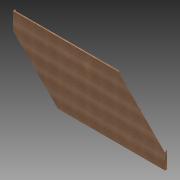
# Autodesk Inventor part: Base
Saved by Autodesk Inventor 2014 SP1 (Build 180222100, 222)
## iProperties
Created: 2015-03-28
Part Number: Base
Material: Wood (Birch)
Document SubType Name: Modeling
Designer: tuleu
Density: 0.55 g/cm^3
Appearance: Birch - Natural Polished
Author: tuleu
Autodesk Inventor part; units mm, degrees
ref_plane "YZ Plane" through (0, 0, 0) normal (1, 0, 0) x (0, 1, 0)
ref_plane "XZ Plane" through (0, 0, 0) normal (0, 1, 0) x (-1, 0, 0)
ref_plane "XY Plane" through (0, 0, 0) normal (0, 0, 1) x (1, 0, 0)
sketch "Sketch1" plane through (0, 0, 0) normal (0, 1, 0) x (-1, 0, 0)
  line L0 (1400, 575) -> (-1400, 575)
  line L1 (-1400, 575) -> (-1400, -575)
  line L2 (-1400, -575) -> (1400, -575)
  line L3 (1400, -575) -> (1400, 575)
  line L4 (0, -575) -> (0, 575)
  line L5 (-1400, 0) -> (1400, 0)
  point P0 (0, 0)
  dimension "d0" = 2800
  dimension "d1" = 1150
  constraints: 12 end point, 6 midpoint, 2 parallel, 1 horizontal, 1 perpendicular
  measures "d0" distance of L1.end L2.end
  measures "d1" distance of L2.end L0.start
extrude "Extrusion1" add sketch "Sketch1" along normal blind 19
sketch "Sketch2" plane through (0, 19, 0) normal (0, 1, 0) x (1, 0, 0)
  line L0 (1400, 575) -> (-1400, 575) projected
  line L1 (-1400, 575) -> (-1400, -575) projected
  line L2 (-1400, -575) -> (1400, -575) projected
  line L3 (1400, -575) -> (1400, 575) projected
  line L4 (-1385, -575) -> (-1385, 575)
  line L5 (1385, 575) -> (1385, -575)
  line L6 (-1385, -575) -> (-1400, -575)
  line L7 (-1400, 575) -> (-1400, -575)
  line L8 (1400, 575) -> (1400, -575)
  line L9 (1400, -575) -> (1385, -575)
  line L10 (-1400, 575) -> (-1385, 575)
  line L11 (1385, 575) -> (1400, 575)
  point P0 (0, 0)
  dimension "d4" = 15
  dimension "d5" = 15
  constraints: 16 end point, 4 perpendicular, 3 collinear, 2 point on line, 1 parallel
  measures "d4" distance between parallel lines of L1 L4
  measures "d5" distance between parallel lines of L3 L5
extrude "Extrusion2" add sketch "Sketch2" along normal blind 19 contours L3 L2 L5 L0 | L4 L2 L1 L0
sketch "Sketch4" plane through (0, 19, 0) normal (0, 1, 0) x (1, 0, 0)
  line L0 (-1385, 575) -> (-1385, -575) projected
  line L1 (-1385, -575) -> (1385, -575) projected
  line L2 (1385, -575) -> (1385, 575) projected
  line L3 (1385, 575) -> (-1385, 575) projected
  line L4 (-1255, -225) -> (-1309.8, -225) projected
  line L5 (-1177.5, 175) -> (-1232.3, 175) projected
  line L6 (-1275, 475) -> (-1385, 475) projected
  line L7 (-1165, 475) -> (-1270, 475) projected
  line L8 (-1060, 475) -> (-1160, 475) projected
  line L9 (-950, 475) -> (-1055, 475) projected
  line L10 (-835, 475) -> (-945, 475) projected
  line L11 (-735, 475) -> (-830, 475) projected
  line L12 (-625, 475) -> (-730, 475) projected
  line L13 (-520, 475) -> (-620, 475) projected
  line L14 (-410, 475) -> (-515, 475) projected
  line L15 (-305, 475) -> (-405, 475) projected
  line L16 (-195, 475) -> (-300, 475) projected
  line L17 (-95, 475) -> (-190, 475) projected
  line L18 (20, 475) -> (-90, 475) projected
  line L19 (130, 475) -> (25, 475) projected
  line L20 (235, 475) -> (135, 475) projected
  line L21 (345, 475) -> (240, 475) projected
  line L22 (460, 475) -> (350, 475) projected
  line L23 (560, 475) -> (465, 475) projected
  line L24 (670, 475) -> (565, 475) projected
  line L25 (775, 475) -> (675, 475) projected
  line L26 (885, 475) -> (780, 475) projected
  line L27 (990, 475) -> (890, 475) projected
  line L28 (1100, 475) -> (995, 475) projected
  line L29 (1200, 475) -> (1105, 475) projected
  line L30 (1385, 475) -> (1205, 475) projected
  line L31 (0, 575) -> (0, 475)
  line L32 (-1385, 525) -> (1385, 525)
  line L33 (-1332.5, 542.5) -> (1297.5, 542.5)
  line L34 (-1330, 475) -> (-1330, -575)
  line L35 (-1217.5, 475) -> (-1217.5, -575)
  line L36 (-1110, 475) -> (-1110, -575)
  line L37 (-1002.5, 475) -> (-1002.5, -575)
  line L38 (-890, 475) -> (-890, -575)
  line L39 (-782.5, 475) -> (-782.5, -575)
  line L40 (-677.5, 475) -> (-677.5, -575)
  line L41 (-570, 475) -> (-570, -575)
  line L42 (-462.5, 475) -> (-462.5, -575)
  line L43 (-355, 475) -> (-355, -575)
  line L44 (-247.5, 475) -> (-247.5, -575)
  line L45 (-142.5, 475) -> (-142.5, -575)
  line L46 (-35, 475) -> (-35, -575)
  line L47 (77.5, 475) -> (77.5, -575)
  line L48 (185, 475) -> (185, -575)
  line L49 (292.5, 475) -> (292.5, -575)
  line L50 (405, 475) -> (405, -575)
  line L51 (512.5, 475) -> (512.5, -575)
  line L52 (617.5, 475) -> (617.5, -575)
  line L53 (725, 475) -> (725, -575)
  line L54 (832.5, 475) -> (832.5, -575)
  line L55 (940, 475) -> (940, -575)
  line L56 (1047.5, 475) -> (1047.5, -575)
  line L57 (1152.5, 475) -> (1152.5, -575)
  line L58 (1295, 475) -> (1295, -575)
  line L59 (-780, 507.5) -> (-780, -195)
  line L60 (-780, -205) -> (-785, -205)
  line L61 (-785, -205) -> (-785, 507.5)
  line L62 (-675, 507.5) -> (-675, 205)
  line L63 (-675, 195) -> (-680, 195)
  line L64 (-680, 205) -> (-680, 507.5)
  line L65 (-567.5, 507.5) -> (-567.5, -195)
  line L66 (-567.5, -205) -> (-572.5, -205)
  line L67 (-572.5, -195) -> (-572.5, 507.5)
  line L68 (-460, 507.5) -> (-460, 205)
  line L69 (-460, 195) -> (-465, 195)
  line L70 (-465, 205) -> (-465, 507.5)
  line L71 (-352.5, 507.5) -> (-352.5, -195)
  line L72 (-352.5, -205) -> (-357.5, -205)
  line L73 (-357.5, -195) -> (-357.5, 507.5)
  line L74 (-245, 507.5) -> (-245, 205)
  line L75 (-245, 195) -> (-250, 195)
  line L76 (-250, 205) -> (-250, 507.5)
  line L77 (-140, 507.5) -> (-140, -205)
  line L78 (-140, -205) -> (-145, -205)
  line L79 (-145, -195) -> (-145, 507.5)
  line L80 (-1327.5, 507.5) -> (-1327.5, -195)
  line L81 (-1327.5, -205) -> (-1332.5, -205)
  line L82 (-1332.5, -205) -> (-1332.5, 542.5)
  line L83 (-1215, 507.5) -> (-1215, 205)
  line L84 (-1215, 195) -> (-1220, 195)
  line L85 (-1220, 205) -> (-1220, 507.5)
  line L86 (-1107.5, 507.5) -> (-1107.5, -195)
  line L87 (-1107.5, -205) -> (-1112.5, -205)
  line L88 (-1112.5, -195) -> (-1112.5, 507.5)
  line L89 (-1000, 507.5) -> (-1000, 205)
  line L90 (-1000, 195) -> (-1005, 195)
  line L91 (-1005, 205) -> (-1005, 507.5)
  line L92 (-887.5, 507.5) -> (-887.5, -205)
  line L93 (-887.5, -205) -> (-892.5, -205)
  line L94 (-892.5, -195) -> (-892.5, 507.5)
  line L95 (-32.5, 507.5) -> (-32.5, -195)
  line L96 (-32.5, -205) -> (-37.5, -205)
  line L97 (-37.5, -205) -> (-37.5, 507.5)
  line L98 (80, 507.5) -> (80, 205)
  line L99 (80, 195) -> (75, 195)
  line L100 (75, 205) -> (75, 507.5)
  line L101 (-1220, 507.5) -> (-1327.5, 507.5)
  line L102 (-1112.5, 507.5) -> (-1215, 507.5)
  line L103 (-1005, 507.5) -> (-1107.5, 507.5)
  line L104 (-892.5, 507.5) -> (-1000, 507.5)
  line L105 (-785, 507.5) -> (-887.5, 507.5)
  line L106 (-680, 507.5) -> (-780, 507.5)
  line L107 (-572.5, 507.5) -> (-675, 507.5)
  line L108 (-465, 507.5) -> (-567.5, 507.5)
  line L109 (-357.5, 507.5) -> (-460, 507.5)
  line L110 (-250, 507.5) -> (-352.5, 507.5)
  line L111 (-145, 507.5) -> (-245, 507.5)
  line L112 (-37.5, 507.5) -> (-140, 507.5)
  line L113 (75, 507.5) -> (-32.5, 507.5)
  line L114 (-1385, -205) -> (1385, -205)
  line L115 (187.5, 507.5) -> (187.5, -195)
  line L116 (187.5, -205) -> (182.5, -205)
  line L117 (182.5, -195) -> (182.5, 507.5)
  line L118 (295, 507.5) -> (295, 205)
  line L119 (295, 195) -> (290, 195)
  line L120 (290, 205) -> (290, 507.5)
  line L121 (407.5, 507.5) -> (407.5, -205)
  line L122 (407.5, -205) -> (402.5, -205)
  line L123 (402.5, -195) -> (402.5, 507.5)
  line L124 (515, 507.5) -> (515, -195)
  line L125 (515, -205) -> (510, -205)
  line L126 (510, -205) -> (510, 507.5)
  line L127 (620, 507.5) -> (620, 205)
  line L128 (620, 195) -> (615, 195)
  line L129 (615, 205) -> (615, 507.5)
  line L130 (727.5, 507.5) -> (727.5, -195)
  line L131 (727.5, -205) -> (722.5, -205)
  line L132 (722.5, -205) -> (722.5, 507.5)
  line L133 (835, 507.5) -> (835, 205)
  line L134 (835, 195) -> (830, 195)
  line L135 (830, 205) -> (830, 507.5)
  line L136 (942.5, 507.5) -> (942.5, -195)
  line L137 (942.5, -205) -> (937.5, -205)
  line L138 (937.5, -195) -> (937.5, 507.5)
  line L139 (1050, 507.5) -> (1050, 205)
  line L140 (1050, 195) -> (1045, 195)
  line L141 (1045, 205) -> (1045, 507.5)
  line L142 (1155, 507.5) -> (1155, -205)
  line L143 (1155, -205) -> (1150, -205)
  line L144 (1150, -195) -> (1150, 507.5)
  line L145 (182.5, 507.5) -> (80, 507.5)
  line L146 (290, 507.5) -> (187.5, 507.5)
  line L147 (402.5, 507.5) -> (295, 507.5)
  line L148 (510, 507.5) -> (407.5, 507.5)
  line L149 (615, 507.5) -> (515, 507.5)
  line L150 (722.5, 507.5) -> (620, 507.5)
  line L151 (830, 507.5) -> (727.5, 507.5)
  line L152 (937.5, 507.5) -> (835, 507.5)
  line L153 (1045, 507.5) -> (942.5, 507.5)
  line L154 (1150, 507.5) -> (1050, 507.5)
  line L155 (1292.5, 507.5) -> (1155, 507.5)
  line L156 (1297.5, 542.5) -> (1297.5, -195)
  line L157 (1297.5, -205) -> (1292.5, -205)
  line L158 (1292.5, -195) -> (1292.5, 507.5)
  line L159 (-1385, 195) -> (1385, 195)
  line L160 (-1327.5, -195) -> (-1262.5, -195)
  line L161 (-1262.5, -195) -> (-1262.5, -205)
  line L162 (-1262.5, -205) -> (-1327.5, -205)
  line L163 (-1280.2, -200) -> (-1280.2, -225) projected
  line L164 (-1309.8, -250) -> (-1309.8, -200) projected
  line L165 (-1309.8, -200) -> (-1280.2, -200)
  line L166 (-1295, -200) -> (-1295, -195)
  line L167 (-1220, 205) -> (-1245, 205)
  line L168 (-1245, 205) -> (-1245, 195)
  line L169 (-1245, 195) -> (-1220, 195)
  line L170 (-1215, 205) -> (-1190, 205)
  line L171 (-1190, 205) -> (-1190, 195)
  line L172 (-1190, 195) -> (-1215, 195)
  line L173 (-1112.5, -195) -> (-1137.5, -195)
  line L174 (-1137.5, -195) -> (-1137.5, -205)
  line L175 (-1137.5, -205) -> (-1112.5, -205)
  line L176 (-1107.5, -195) -> (-1082.5, -195)
  line L177 (-1082.5, -195) -> (-1082.5, -205)
  line L178 (-1082.5, -205) -> (-1107.5, -205)
  line L179 (-1005, 205) -> (-1030, 205)
  line L180 (-1030, 205) -> (-1030, 195)
  line L181 (-1030, 195) -> (-1005, 195)
  line L182 (-1000, 205) -> (-975, 205)
  line L183 (-975, 205) -> (-975, 195)
  line L184 (-975, 195) -> (-1000, 195)
  line L185 (-892.5, -195) -> (-952.5, -195)
  line L186 (-952.5, -195) -> (-952.5, -205)
  line L187 (-952.5, -205) -> (-892.5, -205)
  line L188 (-952.5, -200) -> (-952.5, -500) projected
  line L189 (-712.5, -225) -> (-712.5, -200) projected
  line L190 (-780, -195) -> (-712.5, -195)
  line L191 (-712.5, -195) -> (-712.5, -205)
  line L192 (-780, -205) -> (-712.5, -205)
  line L193 (-705, 200) -> (-705, -100) projected
  line L194 (-650, 175) -> (-650, 200) projected
  line L195 (-397.5, -200) -> (-397.5, -500) projected
  line L196 (-342.5, -225) -> (-342.5, -200) projected
  line L197 (-212.5, -200) -> (-212.5, -500) projected
  line L198 (-275, 200) -> (-275, -100) projected
  line L199 (-220, 175) -> (-220, 200) projected
  line L200 (27.5, -225) -> (27.5, -200) projected
  line L201 (50, 200) -> (50, -100) projected
  line L202 (105, 175) -> (105, 200) projected
  line L203 (265, 200) -> (265, -100) projected
  line L204 (320, 175) -> (320, 200) projected
  line L205 (157.5, -200) -> (157.5, -500) projected
  line L206 (212.5, -225) -> (212.5, -200) projected
  line L207 (-680, 205) -> (-705, 205)
  line L208 (-705, 205) -> (-705, 195)
  line L209 (-680, 195) -> (-705, 195)
  line L210 (-675, 205) -> (-650, 205)
  line L211 (-650, 205) -> (-650, 195)
  line L212 (-675, 195) -> (-650, 195)
  line L213 (-582.5, -200) -> (-582.5, -500) projected
  line L214 (-527.5, -225) -> (-527.5, -200) projected
  line L215 (-572.5, -195) -> (-582.5, -195)
  line L216 (-582.5, -195) -> (-582.5, -205)
  line L217 (-572.5, -205) -> (-582.5, -205)
  line L218 (-567.5, -195) -> (-527.5, -195)
  line L219 (-527.5, -195) -> (-527.5, -205)
  line L220 (-567.5, -205) -> (-527.5, -205)
  line L221 (-490, 200) -> (-490, -100) projected
  line L222 (-435, 175) -> (-435, 200) projected
  line L223 (342.5, -200) -> (342.5, -500) projected
  line L224 (582.5, -225) -> (582.5, -200) projected
  line L225 (590, 200) -> (590, -100) projected
  line L226 (645, 175) -> (645, 200) projected
  line L227 (712.5, -200) -> (712.5, -500) projected
  line L228 (767.5, -225) -> (767.5, -200) projected
  line L229 (897.5, -200) -> (897.5, -500) projected
  line L230 (952.5, -225) -> (952.5, -200) projected
  line L231 (805, 200) -> (805, -100) projected
  line L232 (860, 175) -> (860, 200) projected
  line L233 (1020, 200) -> (1020, -100) projected
  line L234 (1075, 175) -> (1075, 200) projected
  line L235 (1082.5, -200) -> (1082.5, -500) projected
  line L236 (1267.5, -200) -> (1267.5, -500) projected
  line L237 (1322.5, -225) -> (1322.5, -200) projected
  line L238 (-397.5, -205) -> (-397.5, -195)
  line L239 (-397.5, -195) -> (-357.5, -195)
  line L240 (-352.5, -195) -> (-342.5, -195)
  line L241 (-342.5, -195) -> (-342.5, -205)
  line L242 (-342.5, -205) -> (-352.5, -205)
  line L243 (-357.5, -205) -> (-397.5, -205)
  line L244 (-145, -195) -> (-212.5, -195)
  line L245 (-212.5, -195) -> (-212.5, -205)
  line L246 (-212.5, -205) -> (-145, -205)
  line L247 (-465, 205) -> (-490, 205)
  line L248 (-490, 205) -> (-490, 195)
  line L249 (-490, 195) -> (-465, 195)
  line L250 (-460, 205) -> (-435, 205)
  line L251 (-435, 205) -> (-435, 195)
  line L252 (-435, 195) -> (-460, 195)
  line L253 (-250, 205) -> (-275, 205)
  line L254 (-275, 205) -> (-275, 195)
  line L255 (-275, 195) -> (-250, 195)
  line L256 (-245, 195) -> (-220, 195)
  line L257 (-220, 205) -> (-245, 205)
  line L258 (-220, 205) -> (-220, 195)
  line L259 (75, 205) -> (50, 205)
  line L260 (50, 205) -> (50, 195)
  line L261 (50, 195) -> (75, 195)
  line L262 (80, 195) -> (105, 195)
  line L263 (105, 195) -> (105, 205)
  line L264 (105, 205) -> (80, 205)
  line L265 (290, 205) -> (265, 205)
  line L266 (265, 205) -> (265, 195)
  line L267 (265, 195) -> (290, 195)
  line L268 (295, 195) -> (320, 195)
  line L269 (320, 195) -> (320, 205)
  line L270 (320, 205) -> (295, 205)
  line L271 (620, 205) -> (645, 205)
  line L272 (645, 205) -> (645, 195)
  line L273 (675, 195) -> (620, 195)
  line L274 (615, 195) -> (590, 195)
  line L275 (590, 195) -> (590, 205)
  line L276 (590, 205) -> (615, 205)
  line L277 (835, 205) -> (805, 205)
  line L278 (805, 205) -> (805, 195)
  line L279 (805, 195) -> (830, 195)
  line L280 (835, 195) -> (860, 195)
  line L281 (860, 195) -> (860, 205)
  line L282 (860, 205) -> (835, 205)
  line L283 (1020, 195) -> (1020, 205)
  line L284 (1045, 205) -> (1020, 205)
  line L285 (1050, 205) -> (1075, 205)
  line L286 (1075, 205) -> (1075, 195)
  line L287 (-32.5, -195) -> (27.5, -195)
  line L288 (27.5, -195) -> (27.5, -205)
  line L289 (27.5, -205) -> (-32.5, -205)
  line L290 (182.5, -195) -> (157.5, -195)
  line L291 (157.5, -195) -> (157.5, -205)
  line L292 (157.5, -205) -> (182.5, -205)
  line L293 (187.5, -205) -> (212.5, -205)
  line L294 (212.5, -205) -> (212.5, -195)
  line L295 (212.5, -195) -> (187.5, -195)
  line L296 (402.5, -195) -> (342.5, -195)
  line L297 (342.5, -195) -> (342.5, -205)
  line L298 (342.5, -205) -> (402.5, -205)
  line L299 (515, -195) -> (582.5, -195)
  line L300 (582.5, -195) -> (582.5, -205)
  line L301 (582.5, -205) -> (515, -205)
  line L302 (727.5, -195) -> (767.5, -195)
  line L303 (767.5, -205) -> (767.5, -195)
  line L304 (767.5, -205) -> (727.5, -205)
  line L305 (937.5, -195) -> (897.5, -195)
  line L306 (897.5, -205) -> (897.5, -195)
  line L307 (897.5, -205) -> (937.5, -205)
  line L308 (942.5, -205) -> (952.5, -205)
  line L309 (952.5, -205) -> (952.5, -195)
  line L310 (952.5, -195) -> (942.5, -195)
  line L311 (1150, -195) -> (1082.5, -195)
  line L312 (1082.5, -195) -> (1082.5, -205)
  line L313 (1082.5, -205) -> (1150, -205)
  line L314 (1292.5, -195) -> (1267.5, -195)
  line L315 (1267.5, -195) -> (1267.5, -205)
  line L316 (1267.5, -205) -> (1292.5, -205)
  line L317 (1297.5, -195) -> (1322.5, -195)
  line L318 (1322.5, -195) -> (1322.5, -205)
  line L319 (1322.5, -205) -> (1297.5, -205)
  point P0 (0, 0)
  point P1 (0, 525)
  dimension "d11" = 20
  dimension "d12" = 35
  dimension "d13" = 5
  dimension "d14" = 20
  dimension "d17" = 10
  dimension "d18" = 5
  dimension "d19" = 55
  dimension "d20" = 5
  dimension "d21" = 5
  dimension "d22" = 5
  dimension "d23" = 5
  dimension "d24" = 5
  dimension "d25" = 5
  dimension "d26" = 5
  dimension "d27" = 5
  dimension "d28" = 5
  dimension "d29" = 5
  dimension "d30" = 5
  dimension "d31" = 5
  dimension "d32" = 5
  dimension "d33" = 5
  dimension "d34" = 5
  dimension "d35" = 5
  dimension "d36" = 5
  dimension "d37" = 5
  dimension "d38" = 5
  dimension "d39" = 5
  dimension "d40" = 5
  dimension "d41" = 5
  dimension "d42" = 5
  constraints: 500 end point, 110 collinear, 72 parallel, 50 perpendicular, 41 vertical, 39 equal length, 33 horizontal, 30 midpoint, 8 point on line, 104 other
  measures "d12" distance between parallel lines of L101 L33
  measures "d13" distance between parallel lines of L82 L80
  measures "d17" distance between parallel lines of L162 L160
  measures "d18" distance between parallel lines of L83 L85
  measures "d19" distance between parallel lines of L168 L171
  measures "d20" distance between parallel lines of L86 L88
  measures "d21" distance between parallel lines of L89 L91
  measures "d22" distance between parallel lines of L92 L94
  measures "d23" distance between parallel lines of L59 L61
  measures "d24" distance between parallel lines of L64 L62
  measures "d25" distance between parallel lines of L65 L67
  measures "d26" distance between parallel lines of L68 L70
  measures "d27" distance between parallel lines of L73 L71
  measures "d28" distance between parallel lines of L77 L79
  measures "d29" distance between parallel lines of L74 L76
  measures "d30" distance between parallel lines of L95 L97
  measures "d31" distance between parallel lines of L98 L100
  measures "d32" distance between parallel lines of L118 L120
  measures "d33" distance between parallel lines of L127 L129
  measures "d34" distance between parallel lines of L133 L135
  measures "d35" distance between parallel lines of L141 L139
  measures "d36" distance between parallel lines of L115 L117
  measures "d37" distance between parallel lines of L121 L123
  measures "d38" distance between parallel lines of L124 L126
  measures "d39" distance between parallel lines of L130 L132
  measures "d40" distance between parallel lines of L136 L138
  measures "d41" distance between parallel lines of L142 L144
  measures "d42" distance between parallel lines of L156 L158
extrude "Extrusion3" cut sketch "Sketch4" against normal blind 1.5 contours L32 L82 L6 L0 | L6 L82 L159 L0 | L32 L31 L113 L95 L18 L97 L112 L77 L17 L79 L111 L74 L16 L76 L110 L71 L15 L73 L109 L68 L14 L70 L108 L65 L13 L67 L107 L62 L12 L64 L106 L59 L11 L61 L105 L92 L10 L94 L104 L89 L9 L91 L103 L86 L8 L88 L102 L83 L7 L85 L101 L80 L6 L82 | L6 L34 L159 L82 | L32 L156 L30 L158 L155 L142 L29 L144 L154 L139 L28 L141 L153 L136 L27 L138 L152 L133 L26 L135 L151 L130 L25 L132 L150 L127 L24 L129 L149 L124 L23 L126 L148 L121 L22 L123 L147 L118 L21 L120 L146 L115 L20 L117 L145 L98 L19 L100 L113 L31 | L2 L30 L156 L32 | L6 L80 L159 L34 | L2 L159 L156 L30 | L80 L101 L85 L167 L168 L159 | L156 L159 L58 L30 | L2 L114 L237 L318 L317 L156 L159 | L95 L159 L46 L18 | L19 L47 L99 L159 L201 L260 L259 L100 | L58 L159 L158 L30 | L156 L317 L318 L237 L114 L58 L159 | L168 L167 L85 L7 L35 L84 L159 | L46 L159 L97 L18 | L95 L287 L288 L200 L114 L96 L46 L159 | L19 L98 L264 L263 L202 L159 L99 L47 | L58 L114 L236 L315 L314 L158 L159 | L46 L96 L97 L159 | L87 L114 L174 L173 L88 L159 L36 | L36 L159 L86 L176 L177 L114 L87 | L35 L7 L83 L170 L171 L159 L84 | L159 L57 L29 L142 | L142 L114 L57 L159 | L159 L88 L8 L36 | L36 L8 L86 L159 | L159 L45 L17 L77 | L77 L78 L45 L159 | L205 L291 L290 L117 L159 L48 L114 | L159 L144 L29 L57 | L57 L114 L235 L312 L311 L144 L159 | L93 L114 L186 L185 L94 L159 L38 | L38 L159 L92 L93 | L90 L159 L180 L179 L91 L9 L37 | L37 L9 L89 L182 L183 L159 L90 | L159 L79 L17 L45 | L45 L78 L114 L197 L245 L244 L79 L159 | L20 L48 L159 L117 | L60 L61 L159 L39 | L39 L159 L59 L190 L191 L189 L114 L60 | L159 L94 L10 L38 | L38 L10 L92 L159 | L92 L159 L61 L114 | L20 L115 L159 L48 | L48 L159 L115 L295 L294 L206 L114 | L159 L140 L56 L28 L139 L285 L286 L234 | L114 L229 L306 L305 L138 L159 L55 | L55 L159 L136 L310 L309 L230 L114 | L140 L159 L233 L283 L284 L141 L28 L56 | L159 L61 L11 L39 | L39 L11 L59 L159 | L92 L105 L61 L159 | L159 L75 L44 L16 L74 L257 L258 L199 | L159 L138 L27 L55 | L55 L27 L136 L159 | L66 L114 L213 L216 L215 L67 L159 L41 | L41 L159 L65 L218 L219 L214 L114 L66 | L63 L159 L193 L208 L207 L64 L12 L40 | L40 L12 L62 L210 L211 L194 L159 L63 | L72 L114 L195 L238 L239 L73 L159 L43 | L43 L159 L71 L240 L241 L196 L114 L72 | L75 L159 L198 L254 L253 L76 L16 L44 | L114 L223 L297 L296 L123 L159 L50 | L50 L159 L121 L114 | L119 L159 L203 L266 L265 L120 L21 L49 | L49 L21 L118 L270 L269 L204 L159 L119 | L114 L132 L159 L53 | L53 L159 L130 L302 L303 L228 L114 | L159 L67 L13 L41 | L41 L13 L65 L159 | L159 L73 L15 L43 | L43 L15 L71 L159 | L114 L126 L159 L51 | L51 L159 L124 L299 L300 L224 L114 | L159 L123 L22 L50 | L50 L22 L121 L159 | L159 L132 L25 L53 | L53 L25 L130 L159 | L277 L135 L26 L54 | L54 L26 L133 L277 | L69 L159 L221 L248 L247 L70 L14 L42 | L42 L14 L68 L250 L251 L222 L159 L69 | L159 L126 L23 L51 | L51 L23 L124 L159 | L128 L159 L225 L275 L276 L129 L24 L52 | L52 L24 L127 L271 L272 L226 L159 L128
body "Solid1"
